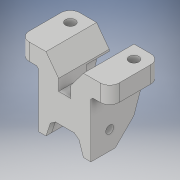
# Autodesk Inventor part: holder-GT2-x-carriage-left
Saved by Autodesk Inventor 2018 (Build 220112000, 112)
## iProperties
Created: 2017-10-15
Part Number: holder-GT2-x-carriage-left
Material: Generic
Document SubType Name: Modeling
Designer: Jurjen
Density: 1 g/cm^3
Appearance: Default
Author: Jurjen
Autodesk Inventor part; units mm, degrees
ref_plane "YZ Plane" through (0, 0, 0) normal (1, 0, 0) x (0, 1, 0)
ref_plane "XZ Plane" through (0, 0, 0) normal (0, 1, 0) x (-1, 0, 0)
ref_plane "XY Plane" through (0, 0, 0) normal (0, 0, 1) x (1, 0, 0)
sketch "Sketch1" plane through (0, 0, 0) normal (0, 0, 1) x (1, 0, 0)
  line L0 (-24, 24) -> (24, 24)
  line L1 (24, 24) -> (24, 15)
  line L2 (24, 15) -> (14, 15)
  line L3 (14, 15) -> (14, -15)
  line L4 (14, -15) -> (10, -15)
  line L5 (10, -15) -> (10, 15)
  line L6 (10, 15) -> (-10, 15)
  line L7 (-10, 15) -> (-10, -15)
  line L8 (-10, -15) -> (-14, -15)
  line L9 (-14, -15) -> (-14, 15)
  line L10 (-14, 15) -> (-24, 15)
  line L11 (-24, 15) -> (-24, 24)
  point P0 (0, 0)
  point P1 (0, 24)
  point P2 (0, 15)
  point P3 (10, 0)
  dimension "d0" = 20
  dimension "d1" = 30
  dimension "d2" = 4
  dimension "d3" = 4
  dimension "d4" = 10
  dimension "d5" = 9
  constraints: 24 end point, 8 perpendicular, 6 point on line, 3 midpoint, 2 vertical alignment, 1 horizontal, 1 horizontal alignment
  measures "d0" distance between parallel lines of L5 L7
  measures "d1" distance between parallel lines of L2 L4
  measures "d2" distance between parallel lines of L3 L5
  measures "d3" distance between parallel lines of L7 L9
  measures "d4" distance between parallel lines of L11 L9
  measures "d5" distance between parallel lines of L0 L2
extrude "Extrusion1" add sketch "Sketch1" along normal mid plane 27
sketch "Sketch2" plane through (-24, 24, 13.5) normal (0, 1, 0) x (1, 0, 0)
  circle A0 centre (7, 20) radius 2.6
  circle A1 centre (41, 20) radius 2.6
  line L0 (0, 27) -> (0, 0) projected
  line L1 (48, 0) -> (48, 27) projected
  line L2 (0, 27) -> (48, 27) projected
  point P0 (24, 13.5)
  dimension "d8" = 5.2
  dimension "d9" = 7
  dimension "d10" = 7
  dimension "d52" = 7
  constraints: 2 centre point, 1 equal radius, 1 horizontal alignment
  measures "d8" diameter of A0
  measures "d9" distance from line of L0 A0.centre
  measures "d10" distance from line of A1.centre L1
  measures "d52" distance from line of A0.centre L2
extrude "Extrusion2" cut sketch "Sketch2" against normal up to next
sketch "Sketch3" plane through (-24, 15, 13.5) normal (0, -1, 0) x (1, 0, 0)
  circle A0 centre (7, -20) radius 2.6 projected
  circle A1 centre (41, -20) radius 2.6 projected
  line L0 (2.85, -22.76) -> (2.85, -17.24)
  line L1 (2.85, -17.24) -> (7, -15.5)
  line L2 (7, -15.5) -> (11.15, -17.24)
  line L3 (11.15, -17.24) -> (11.15, -22.76)
  line L4 (10, 0) -> (10, -27) projected
  line L5 (11.15, -22.76) -> (7, -24.5)
  line L6 (7, -24.5) -> (2.85, -22.76)
  point P0 (24, -13.5)
  point P1 (2.85, -20)
  dimension "d13" = 8.3
  dimension "d22" = 9
  dimension "d23" = 8.3
  constraints: 12 end point, 3 horizontal alignment, 3 parallel, 3 vertical alignment, 1 midpoint, 1 vertical
  measures "d13" distance between parallel lines of L3 L0
  measures "d22" distance of L1.end L5.end
  measures "d23" distance between parallel lines of L6 L2
extrude "Extrusion3" cut sketch "Sketch3" against normal blind 5 and the other way blind 4 contours A0 | L0 L1 L2 L4 L5 L6 | L4 L2 L3 L5
mirror "Mirror1" about plane through (0, 0, 0) normal (1, 0, 0) of "Extrusion3"
sketch "Sketch4" plane through (14, -15, 13.5) normal (1, 0, 0) x (0, 0, -1)
  circle A0 centre (10, 10) radius 2.1
  line L0 (0, 0) -> (27, 0) projected
  point P0 (13.5, 15)
  point P1 (13.5, 0)
  point P2 (13.5, 0)
  dimension "d24" = 4.2
  dimension "d25" = 10
  constraints: 2 midpoint, 2 vertical alignment, 1 centre point
  measures "d24" diameter of A0
  measures "d25" distance from line of A0.centre L0
extrude "Extrusion4" cut sketch "Sketch4" against normal up to surface (28 mm away)
fillet "Fillet1" radius 5 4 edges at (-24, 19.5, 13.5) (-24, 19.5, -13.5) (24, 19.5, 13.5) (24, 19.5, -13.5)
chamfer "Chamfer1" distance 1 angle 45 6 edges at (-14, 15, 5.1211) (-14, 11, -6.5) (-14, 15, -11.6211) (14, 15, 5.1211) (14, 11, -6.5) (14, 15, -11.6211)
sketch "Sketch8" plane through (0, 0, 13.5) normal (0, 0, 1) x (1, 0, 0)
  line L0 (-10, 15) -> (10, 15)
  line L1 (10, 15) -> (10, -15)
  line L2 (10, -15) -> (-10, -15)
  line L3 (-10, -15) -> (-10, 15)
  point P0 (0, 0)
  constraints: 8 end point, 2 parallel, 1 horizontal, 1 perpendicular
extrude "Extrusion7" add sketch "Sketch8" against normal blind 3
sketch "Sketch9" plane through (0, 0, -13.5) normal (0, 0, -1) x (-1, 0, 0)
  line L0 (-10, 5) -> (10, 5)
  line L1 (10, -15) -> (14, -15) projected
  line L2 (-10, 5) -> (-10, 15)
  line L3 (-10, 15) -> (10, 15)
  line L4 (10, 15) -> (10, 5)
  point P0 (0, 0)
  dimension "d44" = 20
  constraints: 8 end point, 2 perpendicular, 2 vertical alignment, 1 horizontal, 1 vertical
  measures "d44" distance between parallel lines of L1 L0
extrude "Extrusion8" add sketch "Sketch9" against normal up to surface (24 mm away)
sketch "Sketch6" plane through (0, 0, 13.5) normal (0, 0, 1) x (1, 0, 0)
  line L0 (-3.25, 15) -> (3.25, 15)
  line L1 (3.25, 15) -> (10, 24)
  line L2 (24, 24) -> (-24, 24) projected
  line L3 (-3.25, 15) -> (-10, 24)
  line L4 (-10, 24) -> (10, 24)
  line L5 (-14, -15) -> (-10, -15) projected
  line L6 (-10, 5) -> (10, 5) projected
  line L7 (-3.25, 15) -> (-3.25, 9)
  line L8 (-3.25, 9) -> (3.25, 9)
  line L9 (3.25, 9) -> (3.25, 15)
  point P0 (0, 0)
  point P1 (0, 15)
  point P2 (0, 24)
  point P3 (-10, 15)
  point P4 (0, 24)
  point P5 (0, 24)
  dimension "d29" = 6.5
  dimension "d30" = 20
  dimension "d47" = 9
  dimension "d48" = 4
  constraints: 14 end point, 4 midpoint, 3 perpendicular, 2 point on line, 1 coincident, 1 collinear, 1 horizontal, 1 vertical alignment
  measures "d29" distance of L0.start L0.end
  measures "d30" distance of L1.end L3.end
  measures "d47" distance between parallel lines of L2 L0
  measures "d48" distance between parallel lines of L6 L8
extrude "Extrusion5" cut sketch "Sketch6" against normal up to surface (27 mm away)
sketch "Sketch11" plane through (-3.25, 9, 13.5) normal (0, 1, 0) x (1, 0, 0)
  line L0 (13.25, 7.9) -> (13.25, 12.1) projected
  line L1 (17.25, 12.1) -> (17.25, 7.9) projected
  circle A0 centre (3.25, 10) radius 2.1
  point P0 (3.25, 13.5)
  point P1 (17.25, 10)
  dimension "d49" = 4.2
  constraints: 1 centre point, 1 horizontal alignment, 1 midpoint, 1 vertical alignment
  measures "d49" diameter of A0
extrude "Extrusion9" cut sketch "Sketch11" against normal up to next
sketch "Sketch12" plane through (0, 0, -13.5) normal (0, 0, -1) x (-1, 0, 0)
  line L0 (-10, 5) -> (10, 5)
  line L1 (10, 5) -> (10, 14)
  line L2 (10, 14) -> (-10, 14)
  line L3 (-10, 14) -> (-10, 5)
  point P0 (0, 0)
  point P1 (-10, -15)
  point P2 (10, -15)
  dimension "d53" = 9
  constraints: 8 end point, 2 parallel, 2 vertical alignment, 1 coincident, 1 horizontal, 1 perpendicular
  measures "d53" distance between parallel lines of L2 L0
extrude "Extrusion10" cut sketch "Sketch12" against normal blind 12
sketch "Sketch13" plane through (14, -15, 13.5) normal (1, 0, 0) x (0, 0, -1)
  line L0 (3, 0) -> (27, 0) projected
  line L1 (13, 0) -> (27, 14)
  line L2 (27, 29) -> (27, 0) projected
  line L3 (22.9, 9.9) -> (27, 21.5)
  point P0 (13.5, 15)
  dimension "d58" = 45
  dimension "d59" = 14
  dimension "d62" = 7.5
  dimension "d63" = 4.1
  constraints: 4 end point, 4 point on line
  measures "d58" angle of L2 L1
  measures "d59" distance of L0.end L1.end
  measures "d62" distance of L1.end L3.end
  measures "d63" horizontal distance of L1.end L3.start
extrude "Extrusion11" cut sketch "Sketch13" against normal through all
sketch "Sketch14" plane through (0, 0, 13.5) normal (0, 0, 1) x (1, 0, 0)
  line L0 (10, -15) -> (7, -6)
  line L1 (7, -6) -> (-7, -6)
  line L2 (-7, -6) -> (-10, -15)
  line L3 (-14, -15) -> (14, -15) projected
  point P0 (0, 0)
  dimension "d64" = 3
  dimension "d65" = 3
  dimension "d66" = 9
  constraints: 6 end point, 1 horizontal
  measures "d64" horizontal distance of L0.start L0.end
  measures "d65" horizontal distance of L2.end L1.end
  measures "d66" distance between parallel lines of L3 L1
extrude "Extrusion12" cut sketch "Sketch14" against normal up to next
chamfer "Chamfer2" distance 2 angle 45 2 edges at (7, -6, 12) (-7, -6, 12)
equation "\"d3\" = d2"
equation "\"d65\" = d64"
body "Solid1"
